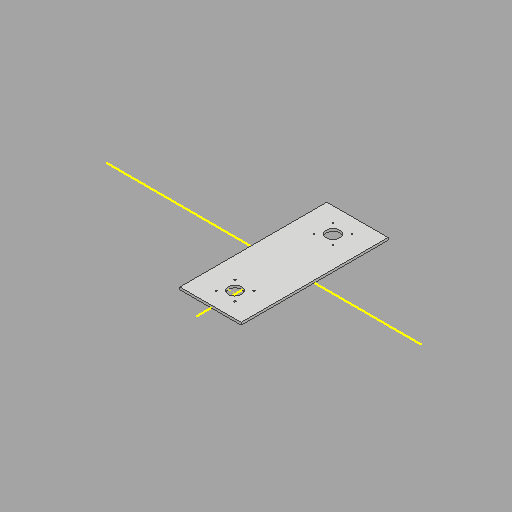
# Autodesk Inventor part: BT001_trajan20_21
Saved by Autodesk Inventor 2022.2 (Build 262287000, 287)
## iProperties
Company: HTBLA Kaindorf
RuleStatus: InUse
Created: 2022-06-05
Part Number: BT001_trajan20_21
Project: Zeichenmaschine_v2
Material: Generisch
Description: Gerüst
Document SubType Name: Modeling
Designer: trajan20
Density: 1 g/cm^3
Appearance: Vorgabe
Mass: 92.807 g
Surface Area: 499.236 cm^2
Volume: 92.807 cm^3
AfterDocNew0: iProperties-Editor_aufrufen
Author: jan
Keywords: 2021
Autodesk Inventor part; units mm, degrees
ref_plane "YZ Plane" through (0, 0, 0) normal (1, 0, 0) x (0, 1, 0)
ref_plane "XZ Plane" through (0, 0, 0) normal (0, 1, 0) x (-1, 0, 0)
ref_plane "XY Plane" through (0, 0, 0) normal (0, 0, 1) x (1, 0, 0)
derived "MS000_trajan20_21_Zeichenmaschine_Inventor_Masterskizze.ipt"
sketch "Skizze16" plane through (110, 40, -80) normal (1, 0, 0) x (0, 1, 0)
  line L0 (-90, 0) -> (10, 0)
  line L1 (10, 0) -> (10, -4)
  line L2 (10, -4) -> (-90, -4)
  line L3 (-90, -4) -> (-90, 0)
  point P0 (-40, 80)
  point P1 (0, 0)
  point P2 (-80, 0)
sketch "Skizze18" plane through (110, -50, -84) normal (0, 0, 1) x (1, 0, 0)
  line L0 (-110, -240.8766) -> (-110, 273.4794)
  line L1 (-134, 50) -> (34, 50)
  line L2 (-14.5, 65.5) -> (-45.5, 65.5) construction
  line L3 (-45.5, 65.5) -> (-45.5, 34.5) construction
  line L4 (-14.5, 65.5) -> (-14.5, 34.5) construction
  line L5 (-14.5, 34.5) -> (-45.5, 34.5) construction
  point P0 (-110, 50)
  point P1 (-30, 50)
  point P2 (-14.5, 65.5)
  point P3 (-14.5, 34.5)
extrude "Extrusion4" add sketch "Skizze16" along normal blind 10 and the other way blind 110
hole "Bohrung4" at (80, 0, -84) direction (0, 0, 1) diameter 22 end through all
hole "Bohrung5" at (64.5, -15.5, -84) at (64.5, 15.5, -84) at (95.5, 15.5, -84) at (95.5, -15.5, -84) direction (0, 0, 1) diameter 2.459 end through all thread size "M3x0.5" class "6H" standard "ISO Metric profile"
mirror "Spiegeln3" about plane through (0, 0, -82) normal (-1, 0, 0)
equation "\"d24\" = 0.5 * Alu_Prof"
equation "\"d25\" = 0.5 * Bas_Haupt_Länge"
equation "\"d35\" = SM_Scheibe_Durchmesser"
equation "\"Alu_Prof\" = 20"
equation "\"Bas_Haupt_Länge\" = 220"
equation "\"SM_Scheibe_Durchmesser\" = 22"
